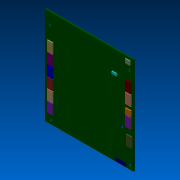
# Autodesk Inventor part: LaunchpadBoard.brd
Saved by Autodesk Inventor 2013 (Build 170138000, 138)
## iProperties
Created: 2014-11-03
Part Number: LaunchpadBoard.brd
Material: Generic
Document SubType Name: Modeling
Designer: Jeramy
Density: 1 g/cm^3
Author: Jeramy
Autodesk Inventor part; units mm, degrees
ref_plane "YZ Plane" through (0, 0, 0) normal (1, 0, 0) x (0, 1, 0)
ref_plane "XZ Plane" through (0, 0, 0) normal (0, 1, 0) x (-1, 0, 0)
ref_plane "XY Plane" through (0, 0, 0) normal (0, 0, 1) x (1, 0, 0)
sketch "Sketch1" plane through (0, 0, 0) normal (0, 0, 1) x (1, 0, 0)
  line L0 (0.508, -0.254) -> (89.662, 0)
  line L1 (89.662, 0) -> (89.662, 97.79)
  line L2 (89.662, 97.79) -> (0.508, 97.79)
  line L3 (0.508, 97.79) -> (0.508, -0.254)
  circle A0 centre (5.08, 86.614) radius 1.6
  circle A1 centre (85.344, 86.868) radius 1.6
  circle A2 centre (85.852, 3.81) radius 1.6
  circle A3 centre (5.842, 3.302) radius 1.6
  circle A4 centre (77.724, 33.274) radius 1.6
  circle A5 centre (81.28, 2.54) radius 0.51
  circle A6 centre (78.74, 2.54) radius 0.51
  circle A7 centre (76.2, 2.54) radius 0.51
  circle A8 centre (73.66, 2.54) radius 0.51
  circle A9 centre (21.34, 2.54) radius 0.51
  circle A10 centre (21.34, 5.08) radius 0.51
  circle A11 centre (21.34, 7.62) radius 0.51
  circle A12 centre (21.34, 10.16) radius 0.51
  circle A13 centre (21.34, 12.7) radius 0.51
  circle A14 centre (21.34, 15.24) radius 0.51
  circle A15 centre (21.34, 17.78) radius 0.51
  circle A16 centre (21.34, 20.32) radius 0.51
  circle A17 centre (21.34, 22.86) radius 0.51
  circle A18 centre (21.34, 25.4) radius 0.51
  circle A19 centre (67.06, 25.4) radius 0.51
  circle A20 centre (67.06, 22.86) radius 0.51
  circle A21 centre (67.06, 20.32) radius 0.51
  circle A22 centre (67.06, 17.78) radius 0.51
  circle A23 centre (67.06, 15.24) radius 0.51
  circle A24 centre (67.06, 12.7) radius 0.51
  circle A25 centre (67.06, 10.16) radius 0.51
  circle A26 centre (67.06, 7.62) radius 0.51
  circle A27 centre (67.06, 5.08) radius 0.51
  circle A28 centre (67.06, 2.54) radius 0.51
  circle A29 centre (23.88, 2.54) radius 0.51
  circle A30 centre (23.88, 5.08) radius 0.51
  circle A31 centre (23.88, 7.62) radius 0.51
  circle A32 centre (23.88, 10.16) radius 0.51
  circle A33 centre (23.88, 12.7) radius 0.51
  circle A34 centre (23.88, 15.24) radius 0.51
  circle A35 centre (23.88, 17.78) radius 0.51
  circle A36 centre (23.88, 20.32) radius 0.51
  circle A37 centre (23.88, 22.86) radius 0.51
  circle A38 centre (23.88, 25.4) radius 0.51
  circle A39 centre (64.52, 25.4) radius 0.51
  circle A40 centre (64.52, 22.86) radius 0.51
  circle A41 centre (64.52, 20.32) radius 0.51
  circle A42 centre (64.52, 17.78) radius 0.51
  circle A43 centre (64.52, 15.24) radius 0.51
  circle A44 centre (64.52, 12.7) radius 0.51
  circle A45 centre (64.52, 10.16) radius 0.51
  circle A46 centre (64.52, 7.62) radius 0.51
  circle A47 centre (64.52, 5.08) radius 0.51
  circle A48 centre (64.52, 2.54) radius 0.51
  circle A49 centre (67.06, 76.71) radius 0.51
  circle A50 centre (67.06, 74.17) radius 0.51
  circle A51 centre (67.06, 71.63) radius 0.51
  circle A52 centre (67.06, 69.09) radius 0.51
  circle A53 centre (67.06, 66.55) radius 0.51
  circle A54 centre (67.06, 64.01) radius 0.51
  circle A55 centre (67.06, 61.47) radius 0.51
  circle A56 centre (67.06, 58.93) radius 0.51
  circle A57 centre (67.06, 56.39) radius 0.51
  circle A58 centre (67.06, 53.85) radius 0.51
  circle A59 centre (21.34, 53.85) radius 0.51
  circle A60 centre (21.34, 56.39) radius 0.51
  circle A61 centre (21.34, 58.93) radius 0.51
  circle A62 centre (21.34, 61.47) radius 0.51
  circle A63 centre (21.34, 64.01) radius 0.51
  circle A64 centre (21.34, 66.55) radius 0.51
  circle A65 centre (21.34, 69.09) radius 0.51
  circle A66 centre (21.34, 71.63) radius 0.51
  circle A67 centre (21.34, 74.17) radius 0.51
  circle A68 centre (21.34, 76.71) radius 0.51
  circle A69 centre (64.52, 76.71) radius 0.51
  circle A70 centre (64.52, 74.17) radius 0.51
  circle A71 centre (64.52, 71.63) radius 0.51
  circle A72 centre (64.52, 69.09) radius 0.51
  circle A73 centre (64.52, 66.55) radius 0.51
  circle A74 centre (64.52, 64.01) radius 0.51
  circle A75 centre (64.52, 61.47) radius 0.51
  circle A76 centre (64.52, 58.93) radius 0.51
  circle A77 centre (64.52, 56.39) radius 0.51
  circle A78 centre (64.52, 53.85) radius 0.51
  circle A79 centre (23.88, 53.85) radius 0.51
  circle A80 centre (23.88, 56.39) radius 0.51
  circle A81 centre (23.88, 58.93) radius 0.51
  circle A82 centre (23.88, 61.47) radius 0.51
  circle A83 centre (23.88, 64.01) radius 0.51
  circle A84 centre (23.88, 66.55) radius 0.51
  circle A85 centre (23.88, 69.09) radius 0.51
  circle A86 centre (23.88, 71.63) radius 0.51
  circle A87 centre (23.88, 74.17) radius 0.51
  circle A88 centre (23.88, 76.71) radius 0.51
  circle A89 centre (6.22, 63.75) radius 0.51
  circle A90 centre (6.48, 66.29) radius 0.51
  circle A91 centre (6.22, 68.83) radius 0.51
  circle A92 centre (6.48, 71.37) radius 0.51
  circle A93 centre (6.22, 53.09) radius 0.51
  circle A94 centre (6.48, 55.63) radius 0.51
  circle A95 centre (6.22, 58.17) radius 0.51
  circle A96 centre (6.48, 60.71) radius 0.51
  circle A97 centre (85.85, 28.7) radius 0.51
  circle A98 centre (85.85, 26.16) radius 0.51
  circle A99 centre (85.85, 23.62) radius 0.51
  circle A100 centre (85.85, 21.08) radius 0.51
  circle A101 centre (84.84, 51.31) radius 0.51
  circle A102 centre (84.84, 48.77) radius 0.51
  circle A103 centre (84.96, 45.21) radius 0.51
  circle A104 centre (84.71, 42.67) radius 0.51
  circle A105 centre (84.96, 40.13) radius 0.51
  circle A106 centre (84.71, 37.59) radius 0.51
  circle A107 centre (84.96, 75.95) radius 0.51
  circle A108 centre (84.71, 73.41) radius 0.51
  circle A109 centre (84.96, 70.87) radius 0.51
  circle A110 centre (84.71, 68.33) radius 0.51
  circle A111 centre (84.96, 65.02) radius 0.51
  circle A112 centre (84.71, 62.48) radius 0.51
  circle A113 centre (84.96, 59.94) radius 0.51
  circle A114 centre (84.71, 57.4) radius 0.51
  circle A115 centre (6.22, 42.42) radius 0.51
  circle A116 centre (6.48, 44.96) radius 0.51
  circle A117 centre (6.22, 47.5) radius 0.51
  circle A118 centre (6.48, 50.04) radius 0.51
  circle A119 centre (6.22, 10.41) radius 0.51
  circle A120 centre (6.48, 12.95) radius 0.51
  circle A121 centre (6.22, 15.49) radius 0.51
  circle A122 centre (6.48, 18.03) radius 0.51
  circle A123 centre (6.22, 31.75) radius 0.51
  circle A124 centre (6.48, 34.29) radius 0.51
  circle A125 centre (6.22, 36.83) radius 0.51
  circle A126 centre (6.48, 39.37) radius 0.51
  circle A127 centre (6.22, 21.08) radius 0.51
  circle A128 centre (6.48, 23.62) radius 0.51
  circle A129 centre (6.22, 26.16) radius 0.51
  circle A130 centre (6.48, 28.7) radius 0.51
  circle A131 centre (79.756, 11.43) radius 0.3
  circle A132 centre (79.502, 23.114) radius 0.3
  circle A133 centre (43.942, 34.544) radius 0.3
  circle A134 centre (81.788, 34.544) radius 0.3
  circle A135 centre (77.978, 26.67) radius 0.3
  circle A136 centre (22.098, 38.862) radius 0.3
  circle A137 centre (14.224, 44.958) radius 0.3
  circle A138 centre (17.526, 43.688) radius 0.3
  circle A139 centre (79.502, 82.55) radius 0.3
  circle A140 centre (30.734, 43.434) radius 0.3
  circle A141 centre (36.322, 8.636) radius 0.3
  circle A142 centre (37.592, 32.766) radius 0.3
  circle A143 centre (32.004, 7.874) radius 0.3
  circle A144 centre (35.814, 34.798) radius 0.3
  circle A145 centre (73.914, 27.178) radius 0.3
  circle A146 centre (36.83, 44.45) radius 0.3
  constraints: 147 centre point, 8 end point
extrude "Launchpad Board.brd_Outline" add sketch "Sketch1" along normal blind 1.6
sketch "1X04, 9D0FSENSORSTICK_1X04_1" plane through (0, 0, 1.6) normal (0, 0, 1) x (1, 0, 0)
  line L0 (82.55, 1.1684) -> (72.39, 1.1684)
  line L1 (72.39, 1.1684) -> (72.39, 3.81)
  line L2 (72.39, 3.81) -> (82.55, 3.81)
  line L3 (82.55, 3.81) -> (82.55, 1.1684)
  constraints: 8 end point
extrude "9D0FSENSORSTICK_2" add sketch "1X04, 9D0FSENSORSTICK_1X04_1" along normal blind 1
sketch "4X10-BOOSTERPACK, A1_4X10-BOOSTERPACK_3" plane through (0, 0, 0) normal (0, 0, 1) x (1, 0, 0)
  line L0 (20.066, 1.27) -> (68.326, 1.27)
  line L1 (68.326, 1.27) -> (68.326, 26.67)
  line L2 (68.326, 26.67) -> (20.066, 26.67)
  line L3 (20.066, 26.67) -> (20.066, 1.27)
  constraints: 8 end point
extrude "A1_4" add sketch "4X10-BOOSTERPACK, A1_4X10-BOOSTERPACK_3" against normal blind 1
sketch "4X10-BOOSTERPACK, A2_4X10-BOOSTERPACK_5" plane through (0, 0, 0) normal (0, 0, 1) x (1, 0, 0)
  line L0 (68.326, 77.978) -> (20.066, 77.978)
  line L1 (20.066, 77.978) -> (20.066, 52.578)
  line L2 (20.066, 52.578) -> (68.326, 52.578)
  line L3 (68.326, 52.578) -> (68.326, 77.978)
  constraints: 8 end point
extrude "A2_6" add sketch "4X10-BOOSTERPACK, A2_4X10-BOOSTERPACK_5" against normal blind 1
sketch "MOLEX-1X4_LOCK, PORTFWD_MOLEX-1X4_LOCK_7" plane through (0, 0, 1.6) normal (0, 0, 1) x (1, 0, 0)
  line L0 (3.2385, 62.4205) -> (3.2385, 72.644)
  line L1 (3.2385, 72.644) -> (8.9535, 72.644)
  line L2 (8.9535, 72.644) -> (8.9535, 62.4205)
  line L3 (8.9535, 62.4205) -> (3.2385, 62.4205)
  constraints: 8 end point
extrude "PORTFWD_8" add sketch "MOLEX-1X4_LOCK, PORTFWD_MOLEX-1X4_LOCK_7" along normal blind 1
sketch "MOLEX-1X4_LOCK, PORTREV_MOLEX-1X4_LOCK_9" plane through (0, 0, 1.6) normal (0, 0, 1) x (1, 0, 0)
  line L0 (3.2385, 51.7525) -> (3.2385, 61.976)
  line L1 (3.2385, 61.976) -> (8.9535, 61.976)
  line L2 (8.9535, 61.976) -> (8.9535, 51.7525)
  line L3 (8.9535, 51.7525) -> (3.2385, 51.7525)
  constraints: 8 end point
extrude "PORTREV_10" add sketch "MOLEX-1X4_LOCK, PORTREV_MOLEX-1X4_LOCK_9" along normal blind 1
sketch "MOLEX-1X4, PRESSURESENSOR_MOLEX-1X4_11" plane through (0, 0, 1.6) normal (0, 0, 1) x (1, 0, 0)
  line L0 (88.9635, 30.0355) -> (88.9635, 19.812)
  line L1 (88.9635, 19.812) -> (83.2485, 19.812)
  line L2 (83.2485, 19.812) -> (83.2485, 30.0355)
  line L3 (83.2485, 30.0355) -> (88.9635, 30.0355)
  constraints: 8 end point
extrude "PRESSURESENSOR_12" add sketch "MOLEX-1X4, PRESSURESENSOR_MOLEX-1X4_11" along normal blind 1
sketch "MOLEX-1X2, M02POLAR_13" plane through (0, 0, 1.6) normal (0, 0, 1) x (1, 0, 0)
  line L0 (87.9475, 52.6415) -> (87.9475, 47.498)
  line L1 (87.9475, 47.498) -> (82.2325, 47.498)
  line L2 (82.2325, 47.498) -> (82.2325, 52.6415)
  line L3 (82.2325, 52.6415) -> (87.9475, 52.6415)
  constraints: 8 end point
extrude "PWR_14" add sketch "MOLEX-1X2, M02POLAR_13" along normal blind 1
sketch "MOLEX-1X4_LOCK, SERIAL_MOLEX-1X4_LOCK_15" plane through (0, 0, 1.6) normal (0, 0, 1) x (1, 0, 0)
  line L0 (87.9475, 46.5455) -> (87.9475, 36.322)
  line L1 (87.9475, 36.322) -> (82.2325, 36.322)
  line L2 (82.2325, 36.322) -> (82.2325, 46.5455)
  line L3 (82.2325, 46.5455) -> (87.9475, 46.5455)
  constraints: 8 end point
extrude "SERIAL_16" add sketch "MOLEX-1X4_LOCK, SERIAL_MOLEX-1X4_LOCK_15" along normal blind 1
sketch "MOLEX-1X4_LOCK, STBDFWD_MOLEX-1X4_LOCK_17" plane through (0, 0, 1.6) normal (0, 0, 1) x (1, 0, 0)
  line L0 (87.9475, 77.2795) -> (87.9475, 67.056)
  line L1 (87.9475, 67.056) -> (82.2325, 67.056)
  line L2 (82.2325, 67.056) -> (82.2325, 77.2795)
  line L3 (82.2325, 77.2795) -> (87.9475, 77.2795)
  constraints: 8 end point
extrude "STBDFWD_18" add sketch "MOLEX-1X4_LOCK, STBDFWD_MOLEX-1X4_LOCK_17" along normal blind 1
sketch "MOLEX-1X4_LOCK, STBDREV_MOLEX-1X4_LOCK_19" plane through (0, 0, 1.6) normal (0, 0, 1) x (1, 0, 0)
  line L0 (87.9475, 66.3575) -> (87.9475, 56.134)
  line L1 (87.9475, 56.134) -> (82.2325, 56.134)
  line L2 (82.2325, 56.134) -> (82.2325, 66.3575)
  line L3 (82.2325, 66.3575) -> (87.9475, 66.3575)
  constraints: 8 end point
extrude "STBDREV_20" add sketch "MOLEX-1X4_LOCK, STBDREV_MOLEX-1X4_LOCK_19" along normal blind 1
sketch "LOGO-ROCKET, U_2_LOGO-ROCKET_21" plane through (0, 0, 1.6) normal (0, 0, 1) x (1, 0, 0)
  line L0 (82.2833, 95.8215) -> (87.0839, 95.8215)
  line L1 (87.0839, 95.8215) -> (87.0839, 91.7829)
  line L2 (87.0839, 91.7829) -> (82.2833, 91.7829)
  line L3 (82.2833, 91.7829) -> (82.2833, 95.8215)
  constraints: 8 end point
extrude "U_2_22" add sketch "LOGO-ROCKET, U_2_LOGO-ROCKET_21" along normal blind 1
sketch "SILK_3V3_TAG, SILK_3V3_TAG_23" plane through (0, 0, 0) normal (0, 0, 1) x (1, 0, 0)
  line L0 (14.732, 1.2827) -> (19.5199, 1.2827)
  line L1 (19.5199, 1.2827) -> (19.5199, 3.556)
  line L2 (19.5199, 3.556) -> (14.732, 3.556)
  line L3 (14.732, 3.556) -> (14.732, 1.2827)
  constraints: 8 end point
extrude "U_3_24" add sketch "SILK_3V3_TAG, SILK_3V3_TAG_23" against normal blind 1
sketch "SILK_3V3_TAG, SILK_3V3_TAG_25" plane through (0, 0, 1.6) normal (0, 0, 1) x (1, 0, 0)
  line L0 (73.406, 75.7047) -> (68.6181, 75.7047)
  line L1 (68.6181, 75.7047) -> (68.6181, 77.978)
  line L2 (68.6181, 77.978) -> (73.406, 77.978)
  line L3 (73.406, 77.978) -> (73.406, 75.7047)
  constraints: 8 end point
extrude "U_4_26" add sketch "SILK_3V3_TAG, SILK_3V3_TAG_25" along normal blind 1
sketch "MOLEX-1X4_LOCK, VERT1_MOLEX-1X4_LOCK_27" plane through (0, 0, 1.6) normal (0, 0, 1) x (1, 0, 0)
  line L0 (3.2385, 41.0845) -> (3.2385, 51.308)
  line L1 (3.2385, 51.308) -> (8.9535, 51.308)
  line L2 (8.9535, 51.308) -> (8.9535, 41.0845)
  line L3 (8.9535, 41.0845) -> (3.2385, 41.0845)
  constraints: 8 end point
extrude "VERT1_28" add sketch "MOLEX-1X4_LOCK, VERT1_MOLEX-1X4_LOCK_27" along normal blind 1
sketch "MOLEX-1X4_LOCK, VERT2_MOLEX-1X4_LOCK_29" plane through (0, 0, 1.6) normal (0, 0, 1) x (1, 0, 0)
  line L0 (3.2385, 9.0805) -> (3.2385, 19.304)
  line L1 (3.2385, 19.304) -> (8.9535, 19.304)
  line L2 (8.9535, 19.304) -> (8.9535, 9.0805)
  line L3 (8.9535, 9.0805) -> (3.2385, 9.0805)
  constraints: 8 end point
extrude "VERT2_30" add sketch "MOLEX-1X4_LOCK, VERT2_MOLEX-1X4_LOCK_29" along normal blind 1
sketch "MOLEX-1X4_LOCK, VERT3_MOLEX-1X4_LOCK_31" plane through (0, 0, 1.6) normal (0, 0, 1) x (1, 0, 0)
  line L0 (3.2385, 30.4165) -> (3.2385, 40.64)
  line L1 (3.2385, 40.64) -> (8.9535, 40.64)
  line L2 (8.9535, 40.64) -> (8.9535, 30.4165)
  line L3 (8.9535, 30.4165) -> (3.2385, 30.4165)
  constraints: 8 end point
extrude "VERT3_32" add sketch "MOLEX-1X4_LOCK, VERT3_MOLEX-1X4_LOCK_31" along normal blind 1
sketch "MOLEX-1X4_LOCK, VERT4_MOLEX-1X4_LOCK_33" plane through (0, 0, 1.6) normal (0, 0, 1) x (1, 0, 0)
  line L0 (3.2385, 19.7485) -> (3.2385, 29.972)
  line L1 (3.2385, 29.972) -> (8.9535, 29.972)
  line L2 (8.9535, 29.972) -> (8.9535, 19.7485)
  line L3 (8.9535, 19.7485) -> (3.2385, 19.7485)
  constraints: 8 end point
extrude "VERT4_34" add sketch "MOLEX-1X4_LOCK, VERT4_MOLEX-1X4_LOCK_33" along normal blind 1
body "Solid1"
